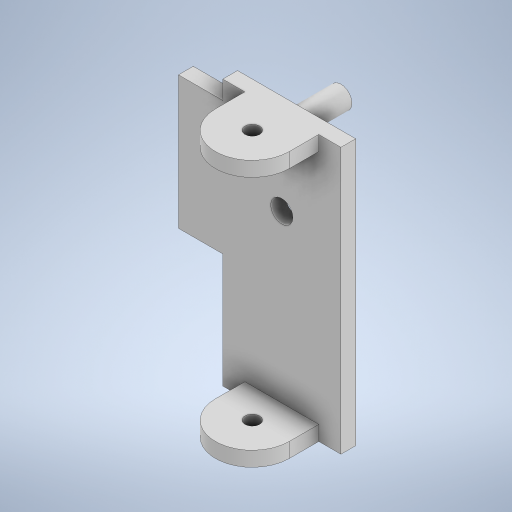
# Autodesk Inventor part: wheel_braket_rear
Saved by Autodesk Inventor 2023 (Build 270158000, 158)
## iProperties
Created: 2024-02-12
Part Number: wheel_braket_rear
Material: 일반
Document SubType Name: Modeling
Designer: ps737
Density: 1 g/cm^3
Appearance: 기본값
Author: ps737
Autodesk Inventor part; units mm, degrees
ref_plane "YZ Plane" through (0, 0, 0) normal (1, 0, 0) x (0, 1, 0)
ref_plane "XZ Plane" through (0, 0, 0) normal (0, 1, 0) x (-1, 0, 0)
ref_plane "XY Plane" through (0, 0, 0) normal (0, 0, 1) x (1, 0, 0)
sketch "스케치1" plane through (0, 0, 0) normal (0, 0, 1) x (1, 0, 0)
  line L0 (80, -122.5) -> (0, -122.5)
  line L1 (0, -122.5) -> (0, 2.5789)
  line L2 (80, 57.5) -> (80, -122.5)
  line L3 (80, -45) -> (80, -122.5)
  line L4 (40, 57.5) -> (40, -122.5)
  circle A0 centre (40, 47.0427) radius 7.5
  circle A1 centre (-7.0427, 0) radius 7.5
  circle A2 centre (40, -47.0427) radius 7.5
  circle A3 centre (87.0427, 0) radius 7.5
  circle A4 centre (40, 0) radius 7.5
  line L5 (0, 57.5) -> (80, 57.5)
  line L6 (0, 45) -> (-30, 45)
  line L7 (-30, 45) -> (-30, -45)
  line L8 (-30, -45) -> (0, -45)
  line L9 (0, 57.5) -> (0, 45)
  point P0 (0, 0)
  point P1 (0, 0)
  dimension "d0" = 80
  dimension "d12" = 15
  dimension "d13" = 360
  dimension "d14" = 0
  dimension "d15" = 47.0427
  dimension "d16" = 47.0427
  dimension "d21" = 15
  dimension "d29" = 122.5
  dimension "d31" = 45
  dimension "d32" = 30
  dimension "d33" = 45
  dimension "d34" = 12.5
  constraints: 20 end point, 4 centre point, 3 perpendicular, 2 coincident, 2 horizontal, 2 midpoint, 2 parallel, 2 point on line, 12 other
  measures "d0" distance of L0.start L0.end
  measures "d12" diameter of A0
  measures "d14" distance from line of L4 A0.centre
  measures "d15" vertical distance of point (0, 0) A0.centre
  measures "d16" vertical distance of point (0, 0) A2.centre
  measures "d21" diameter of A4
  measures "d29" distance from line of L0 point (0, 0)
  measures "d31" distance from line of point (0, 0) L8
  measures "d32" distance between parallel lines of L1 L7
  measures "d33" distance from line of point (0, 0) L6
  measures "d34" distance between parallel lines of L6 L5
extrude "돌출1" add sketch "스케치1" against normal blind 10 contours L0 L4 A2 A4 A0 L5 L2 A3 | L0 L1 L8 L7 L6 L9 L5 L4 A0 A4 A2 | A3 L2 | A4 L4 | L4 A4 | A1 L1 | L1 A1 picked at (79.8647, 0.2918)
extrude "돌출2" add sketch "스케치1" against normal blind 40 contours A2 L4 | L4 A2 | A0 L4 | L4 A0
extrude "돌출3" cut sketch "스케치1" against normal blind 40 contours A4 L4 | L4 A4
sketch "스케치2" plane through (0, -122.5, 0) normal (0, -1, 0) x (1, 0, 0)
  line L0 (0, 0) -> (80, 0) projected
  line L1 (15, 0) -> (15, 20)
  line L2 (15, 20) -> (65, 20)
  line L3 (65, 20) -> (65, 0)
  arc A0 (65, 20) -> (15, 20) centre (40, 20) ccw
  circle A1 centre (40, 20) radius 5
  point P0 (40, 0)
  dimension "d24" = 20
  dimension "d25" = 50
  dimension "d26" = 25
  dimension "d28" = 10
  constraints: 6 end point, 2 centre point, 2 midpoint, 2 perpendicular, 2 point on circle, 2 point on line, 1 coincident, 1 vertical
  measures "d24" distance between parallel lines of L0 L2
  measures "d25" distance between parallel lines of L3 L1
  measures "d26" distance from line of point (40, 0) L1
  measures "d28" diameter of A1
extrude "돌출4" add sketch "스케치2" against normal blind 10 contours L1 L2 A1 L3 L0 | A0 L2 A1
sketch "스케치3" plane through (0, 57.5, 0) normal (0, 1, 0) x (1, 0, 0)
  line L0 (15, 0) -> (15, -20) projected
  arc A0 (15, -20) -> (65, -20) centre (40, -20) ccw projected
  line L1 (65, -20) -> (65, 0) projected
  line L2 (15, 0) -> (65, 0) projected
  circle A1 centre (40, -20) radius 5 projected
  point P0 (0, 0)
extrude "돌출5" add sketch "스케치3" against normal blind 10
